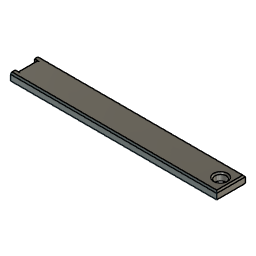
Pixsso_Assembly (Autodesk Fusion 360 archive; units mm, degrees)
design "eInkFrame_BatteryBracket"
Autodesk Fusion 360 part; units mm, degrees
sketch "Sketch1" plane through (0, 0, 0) normal (0, 0, 1) x (1, 0, 0)
  circle A0 centre (0, 0) radius 1.6
  line L0 (3, -4.1) -> (-55.8, -4.1)
  line L1 (-55.8, -4.1) -> (-55.8, 4.1)
  line L2 (-55.8, 4.1) -> (3, 4.1)
  line L3 (3, 4.1) -> (3, -4.1)
  line L4 (3, -4.1) -> (-55.8, 4.1) construction
  line L5 (-55.8, -4.1) -> (3, 4.1) construction
  point P0 (-26.4, 0)
  dimension "d1" = 55.8
  dimension "d2" = 3
  dimension "d3" = 3.2
  dimension "d4" = 8.2
  constraint coincident A0.centre origin
  constraint horizontal L0
  constraint perpendicular L0 L1
  constraint parallel L0 L2
  constraint parallel L1 L3
  constraint coincident L4 P0
  constraint coincident L5 P0
  constraint horizontal A0.centre P0
  measures "d1" distance of A0.centre L1
  measures "d2" distance of A0.centre L3
  measures "d3" diameter of A0
  measures "d4" distance of L0.start L2.end
extrude "Extrude1" add sketch "Sketch1" along normal blind 2
sketch "Sketch2" plane through (0, -4.1, 0) normal (0, -1, 0) x (1, 0, 0)
  line L0 (-55.8, 0) -> (3, 0)
  line L1 (3, 0) -> (3, 2)
  line L2 (3, 2) -> (-55.8, 2)
  line L3 (-55.8, 2) -> (-55.8, 0)
ref_plane "WorkPlane1" through (-26.4, 0, 1) normal (0, 1, 0) x (-1, 0, 0)
sketch "Sketch3" plane through (0, 0, 0) normal (0, 1, 0) x (1, 0, 0)
  line L0 (-55.8, 0) -> (-53.6, -1.2702)
  line L1 (-53.6, -1.2702) -> (-55.8, -2.5403)
  line L2 (-55.8, -2.5403) -> (-55.8, 0)
  line L3 (-55.8, 0) -> (3, 0)
  dimension "d7" = 30
  dimension "d8" = 30
  dimension "d9" = 2.2
  constraint vertical L2
  constraint coincident L0.start L2.end
  measures "d7" angle of L0 L3
  measures "d8" angle of L1 L3
  measures "d9" horizontal distance of L0.end L0.start
extrude "Extrude2" cut sketch "Sketch3" along normal mid plane 5.5
chamfer "Chamfer1" distance 0.4 distance2 0.4 4 edges at (-1.4917, 0.5786, 2) (-26.4, 4.1, 2) (3, 0, 2) (-26.4, -4.1, 2) measured on face at (-37.1094, 0, 2) measured on face at (-37.1094, 0, 2) measured on face at (-37.1094, 0, 2) measured on face at (-37.1094, 0, 2)
